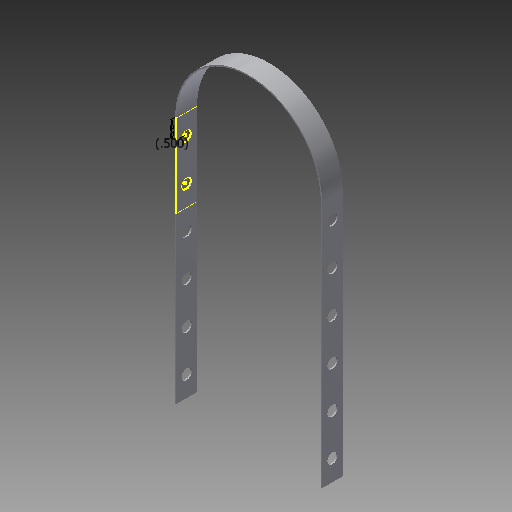
# Autodesk Inventor part: Strap
Saved by Autodesk Inventor 2017 (Build 210142000, 142)
## iProperties
Created: 2016-04-21
Part Number: Strap
Material: Generic
Document SubType Name: Modeling
Designer: Administrator
Density: 1 g/cm^3
Appearance: Aluminum - Flat
Author: Administrator
Autodesk Inventor part; units mm, degrees
ref_plane "YZ Plane" through (0, 0, 0) normal (1, 0, 0) x (0, 1, 0)
ref_plane "XZ Plane" through (0, 0, 0) normal (0, 1, 0) x (-1, 0, 0)
ref_plane "XY Plane" through (0, 0, 0) normal (0, 0, 1) x (1, 0, 0)
sketch "Sketch1" plane through (0, 0, 0) normal (0, 0, 1) x (1, 0, 0)
  line L0 (0, 0) -> (0, 50.8)
  arc A0 (88.9, 50.8) -> (0, 50.8) centre (44.45, 50.8) ccw
  line L1 (88.9, 50.8) -> (88.9, 0)
  line L2 (89.6874, 0) -> (89.6874, 50.8)
  arc A1 (89.6874, 50.8) -> (-0.7874, 50.8) centre (44.45, 50.8) ccw
  line L3 (-0.7874, 50.8) -> (-0.7874, 0)
  line L4 (-0.7874, 50.8) -> (50.0126, 50.8) construction
  line L5 (88.9, 0) -> (88.8999, -101.6)
  line L6 (89.6874, -1.5875) -> (89.6874, -101.6)
  line L7 (89.6874, -101.6) -> (88.8999, -101.6)
  line L8 (-0.7874, 0) -> (-0.7874, -101.6)
  line L9 (0, 0) -> (-0.0001, -101.6)
  line L10 (-0.0001, -101.6) -> (-0.7874, -101.6)
  line L11 (89.6874, 0) -> (89.6874, -1.5875)
  dimension "d1" = 88.9
  dimension "d2" = 44.45
  dimension "d3" = 50.8
  dimension "d5" = 50.8
  dimension "d6" = 90.4748
  dimension "d7" = 45.2374
  dimension "d8" = 50.8
  dimension "d9" = 90
  dimension "d30" = 101.6
  dimension "d32" = 101.6
  constraints: 24 end point, 4 perpendicular, 4 point on circle, 3 parallel, 2 centre point, 2 tangent, 1 horizontal, 1 vertical
  measures "d1" distance of L0.end L1.start
  measures "d2" radius of A0
  measures "d3" distance of L1.start L1.end
  measures "d5" distance of L2.start L2.end
  measures "d6" distance of L2.end L3.start
  measures "d7" radius of A1
  measures "d8" distance of L3.start L3.end
  measures "d9" angle of L3 L4
  measures "d30" distance of L1.end L5.end
  measures "d32" distance of L3.end L8.end
extrude "Extrusion1" add sketch "Sketch1" along normal blind 12.7
hole "Hole1" at (89.6874, 12.7, 6.35) direction (-1, 0, 0) diameter 6.35 end through all
hole "Hole2" at (89.6874, 38.1, 6.35) direction (-1, 0, 0) diameter 6.35 end through all
sketch "Sketch3" plane through (-0.7874, -101.6, 0) normal (-1, 0, 0) x (0, 0, 1)
  line L0 (0, 101.6) -> (12.7, 101.6) projected
  line L1 (6.35, 101.6) -> (6.35, 88.9)
  line L2 (6.35, 88.9) -> (6.35, 63.5)
  dimension "d36" = 12.7
  dimension "d37" = 25.4
  constraints: 4 end point, 2 coincident, 1 collinear, 1 midpoint, 1 perpendicular
  measures "d36" distance of L1.start L1.end
  measures "d37" distance of L2.start L2.end
sketch "Sketch4" plane through (-0.7874, 0, 0) normal (-1, 0, 0) x (0, 0, 1)
  circle A0 centre (6.35, 38.1) radius 3.175 projected
  circle A1 centre (6.35, 12.7) radius 3.175 projected
  line L0 (0, 50.8) -> (0, 0) projected
  line L1 (0, 0) -> (12.7, 0) projected
  line L2 (12.7, 50.8) -> (12.7, 0) projected
  line L3 (0, 50.8) -> (12.7, 50.8) projected
  dimension "d34" = 12.7
  measures "d34" distance from line of L3 A0.centre
hole "Hole3" at (-0.7874, -12.7, 6.35) direction (1, 0, 0) diameter 6.35 end through all
sketch "Sketch5" plane through (-0.7874, -101.6, 0) normal (-1, 0, 0) x (0, 0, 1)
  circle A0 centre (6.35, 88.9) radius 3.175 projected
  line L0 (0, 0) -> (12.7, 0) projected
  line L1 (0, 101.6) -> (12.7, 101.6) projected
  line L2 (6.35, 88.9) -> (6.35, 63.5)
  line L3 (6.35, 88.9) -> (31.75, 88.9) construction
  line L4 (6.35, 63.5) -> (6.35, 38.1)
  line L5 (6.35, 38.1) -> (6.35, 12.7)
  dimension "d45" = 25.4
  dimension "d46" = 90
  dimension "d47" = 25.4
  dimension "d48" = 25.4
  constraints: 8 end point, 3 coincident, 3 perpendicular, 1 collinear, 1 horizontal
  measures "d45" distance of L2.start L2.end
  measures "d46" angle of L2 L3
  measures "d47" distance of L4.start L4.end
  measures "d48" distance of L5.start L5.end
hole "Hole4" at (-0.7874, -38.1, 6.35) direction (1, 0, 0) diameter 6.35 end through all
sketch "Sketch6" plane through (-0.7874, -101.6, 0) normal (-1, 0, 0) x (0, 0, 1)
  circle A0 centre (6.35, 63.5) radius 3.175 projected
  line L0 (0, 101.6) -> (12.7, 101.6) projected
  line L1 (6.35, 63.5) -> (6.35, 38.1)
  dimension "d56" = 25.4
  constraints: 2 end point, 1 coincident, 1 perpendicular
  measures "d56" distance of L1.start L1.end
hole "Hole5" at (-0.7874, -63.5, 6.35) direction (1, 0, 0) diameter 6.35 end through all
sketch "Sketch7" plane through (-0.7874, -101.6, 0) normal (-1, 0, 0) x (0, 0, 1)
  circle A0 centre (6.35, 38.1) radius 3.175 projected
  line L0 (0, 101.6) -> (12.7, 101.6) projected
  line L1 (6.35, 38.1) -> (6.35, 12.7)
  dimension "d64" = 25.4
  constraints: 2 end point, 1 coincident, 1 perpendicular
  measures "d64" distance of L1.start L1.end
hole "Hole6" at (-0.7874, -88.9, 6.35) direction (1, 0, 0) diameter 6.35 end through all
body "Solid1"
